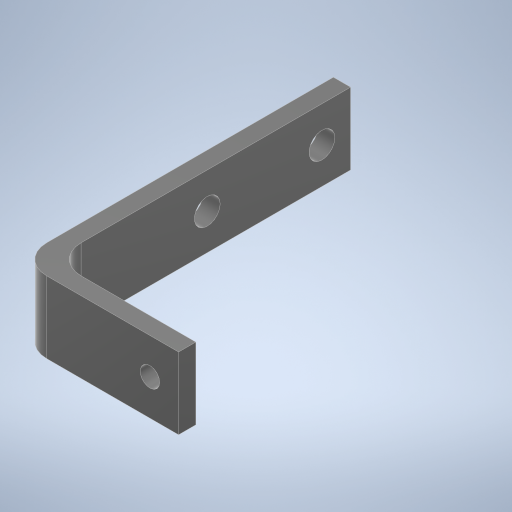
# Autodesk Inventor part: Scissor_fixing_parts
Saved by Autodesk Inventor 2024 (Build 280153000, 153)
## iProperties
Created: 2024-10-12
Part Number: Scissor_fixing_parts
Material: ABS プラスチック
Document SubType Name: Modeling
Designer: 1412z
Density: 1.06 g/cm^3
Appearance: 滑らか - 黒
Author: 1412z
Autodesk Inventor part; units mm, degrees
ref_plane "YZ Plane" through (0, 0, 0) normal (1, 0, 0) x (0, 1, 0)
ref_plane "XZ Plane" through (0, 0, 0) normal (0, 1, 0) x (-1, 0, 0)
ref_plane "XY Plane" through (0, 0, 0) normal (0, 0, 1) x (1, 0, 0)
sketch "スケッチ1" plane through (0, 0, 0) normal (1, 0, 0) x (0, 1, 0)
  line L0 (6.25, -25) -> (-6.25, -25)
  line L1 (-6.25, -25) -> (-6.25, 25)
  line L2 (-6.25, 25) -> (6.25, 25)
  line L3 (6.25, 25) -> (6.25, -25)
  line L4 (6.25, -25) -> (-6.25, 25) construction
  line L5 (-6.25, -25) -> (6.25, 25) construction
  point P0 (0, 0)
  dimension "d0" = 12.5
  dimension "d1" = 50
  constraints: 12 end point, 2 midpoint, 2 parallel, 1 horizontal, 1 perpendicular
  measures "d0" distance of L1.end L2.end
  measures "d1" distance of L0.end L1.end
extrude "押し出し1" add sketch "スケッチ1" along normal mid plane 3
sketch "スケッチ2" plane through (1.5, 0, 0) normal (1, 0, 0) x (0, 0, -1)
  circle A0 centre (20, 0) radius 2.25
  circle A1 centre (0, 0) radius 2.25
  dimension "d4" = 4.5
  dimension "d5" = 4.5
  constraints: 2 centre point, 1 coincident
  measures "d4" diameter of A0
  measures "d5" diameter of A1
extrude "押し出し2" cut sketch "スケッチ2" against normal blind 3
sketch "スケッチ3" plane through (-1.5, -6.25, 25) normal (0, 0, 1) x (1, 0, 0)
  line L0 (0, 0) -> (0, 12.5) projected
  line L1 (3, 12.5) -> (3, 0) projected
  line L2 (0, 0) -> (3, 0)
  line L3 (3, 0) -> (3, 12.5)
  line L4 (3, 12.5) -> (0, 12.5)
  line L5 (0, 12.5) -> (0, 0)
  point P0 (1.5, 6.25)
  constraints: 8 end point, 2 parallel, 1 horizontal, 1 perpendicular
extrude "押し出し3" add sketch "スケッチ3" along normal blind 5
sketch "スケッチ4" plane through (1.5, 0, 0) normal (1, 0, 0) x (0, 0, -1)
  line L0 (25, -6.25) -> (-30, -6.25) projected
  line L1 (25, 6.25) -> (-30, 6.25) projected
  line L2 (-30, -6.25) -> (-27, -6.25)
  line L3 (-27, -6.25) -> (-27, 6.25)
  line L4 (-27, 6.25) -> (-30, 6.25)
  line L5 (-30, 6.25) -> (-30, -6.25)
  point P0 (0, 0)
  dimension "d10" = 3
  constraints: 8 end point, 2 parallel, 1 horizontal, 1 perpendicular, 1 point on line
  measures "d10" distance of L4.end L3.end
extrude "押し出し4" add sketch "スケッチ4" along normal blind 25
fillet "フィレット1" radius 5 1 edges at (1.5, 0, 27)
fillet "フィレット2" radius 5 1 edges at (-1.5, 0, 30)
sketch "スケッチ5" plane through (-1.5, -6.25, 30) normal (0, 0, 1) x (1, 0, 0)
  circle A0 centre (23, 6.25) radius 1.7
  point P0 (1.5, 6.25)
  dimension "d15" = 3.4
  constraints: 1 centre point
  measures "d15" diameter of A0
extrude "押し出し5" cut sketch "スケッチ5" against normal blind 25
